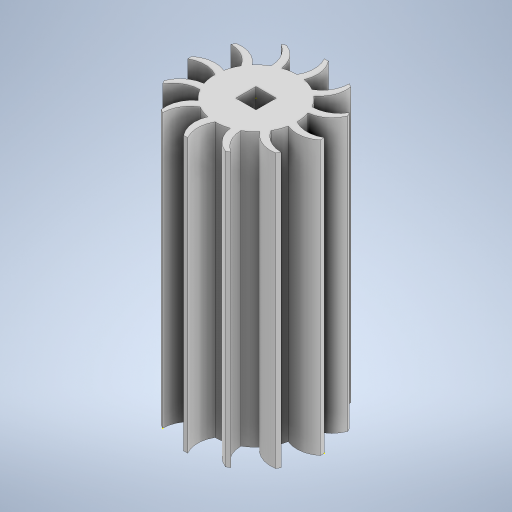
# Autodesk Inventor part: Part4
Saved by Autodesk Inventor 2023 (Build 270158000, 158)
## iProperties
Created: 2024-11-19
Part Number: Part4
Material: Generic
Document SubType Name: Sheet Metal
Designer: 1ZHUSAM
Density: 1 g/cm^3
Sheet Metal Rule: Default_mm
Appearance: Default
Author: 1ZHUSAM
Autodesk Inventor part; units mm, degrees
ref_plane "YZ Plane" through (0, 0, 0) normal (1, 0, 0) x (0, 1, 0)
ref_plane "XZ Plane" through (0, 0, 0) normal (0, 1, 0) x (-1, 0, 0)
ref_plane "XY Plane" through (0, 0, 0) normal (0, 0, 1) x (1, 0, 0)
sketch "Sketch1" plane through (0, 0, 0) normal (0, 1, 0) x (-1, 0, 0)
  circle A0 centre (0, 0) radius 7.5
  line L0 (1.5, 1.5) -> (-1.5, -1.5) construction
  line L1 (-1.5, 1.5) -> (1.5, -1.5) construction
  arc A1 (7.5, 0) -> (12.5, 0) centre (10, 4.3301) ccw
  line L2 (0, 0) -> (5.3033, -5.3033)
  line L3 (0, 0) -> (6.9291, -2.8701)
  line L4 (0, 0) -> (7.5, 0) construction
  line L5 (0, 0) -> (7.3559, -1.4632)
  line L6 (0, 0) -> (7.5, 0) construction
  line L7 (0, 0) -> (7.4639, -0.7351)
  line L8 (0, 0) -> (7.5, 0) construction
  line L9 (12.5, 0) -> (12.5, -0.7351)
  arc A2 (7.4639, -0.7351) -> (7.5, 0) centre (0, 0) ccw
  arc A3 (7.3559, -1.4632) -> (12.5, -0.7351) centre (9.3293, 3.1309) ccw
  arc A4 (6.4952, 3.75) -> (10.8253, 6.25) centre (6.4952, 8.75) ccw
  line L10 (10.8253, 6.25) -> (11.1929, 5.6134)
  arc A5 (7.102, 2.4108) -> (11.1929, 5.6134) centre (6.5139, 7.3761) ccw
  arc A6 (3.75, 6.4952) -> (6.25, 10.8253) centre (1.25, 10.8253) ccw
  line L11 (6.25, 10.8253) -> (6.8866, 10.4578)
  arc A7 (4.9451, 5.6388) -> (6.8866, 10.4578) centre (1.9532, 9.6448) ccw
  arc A8 (0, 7.5) -> (0, 12.5) centre (-4.3301, 10) ccw
  line L12 (0, 12.5) -> (0.7351, 12.5)
  arc A9 (1.4632, 7.3559) -> (0.7351, 12.5) centre (-3.1309, 9.3293) ccw
  arc A10 (-3.75, 6.4952) -> (-6.25, 10.8253) centre (-8.75, 6.4952) ccw
  line L13 (-6.25, 10.8253) -> (-5.6134, 11.1929)
  arc A11 (-2.4108, 7.102) -> (-5.6134, 11.1929) centre (-7.3761, 6.5139) ccw
  arc A12 (-6.4952, 3.75) -> (-10.8253, 6.25) centre (-10.8253, 1.25) ccw
  line L14 (-10.8253, 6.25) -> (-10.4578, 6.8866)
  arc A13 (-5.6388, 4.9451) -> (-10.4578, 6.8866) centre (-9.6448, 1.9532) ccw
  arc A14 (-7.5, 0) -> (-12.5, 0) centre (-10, -4.3301) ccw
  line L15 (-12.5, 0) -> (-12.5, 0.7351)
  arc A15 (-7.3559, 1.4632) -> (-12.5, 0.7351) centre (-9.3293, -3.1309) ccw
  arc A16 (-6.4952, -3.75) -> (-10.8253, -6.25) centre (-6.4952, -8.75) ccw
  line L16 (-10.8253, -6.25) -> (-11.1929, -5.6134)
  arc A17 (-7.102, -2.4108) -> (-11.1929, -5.6134) centre (-6.5139, -7.3761) ccw
  arc A18 (-3.75, -6.4952) -> (-6.25, -10.8253) centre (-1.25, -10.8253) ccw
  line L17 (-6.25, -10.8253) -> (-6.8866, -10.4578)
  arc A19 (-4.9451, -5.6388) -> (-6.8866, -10.4578) centre (-1.9532, -9.6448) ccw
  arc A20 (0, -7.5) -> (0, -12.5) centre (4.3301, -10) ccw
  line L18 (0, -12.5) -> (-0.7351, -12.5)
  arc A21 (-1.4632, -7.3559) -> (-0.7351, -12.5) centre (3.1309, -9.3293) ccw
  arc A22 (3.75, -6.4952) -> (6.25, -10.8253) centre (8.75, -6.4952) ccw
  line L19 (6.25, -10.8253) -> (5.6134, -11.1929)
  arc A23 (2.4108, -7.102) -> (5.6134, -11.1929) centre (7.3761, -6.5139) ccw
  arc A24 (6.4952, -3.75) -> (10.8253, -6.25) centre (10.8253, -1.25) ccw
  line L20 (10.8253, -6.25) -> (10.4578, -6.8866)
  arc A25 (5.6388, -4.9451) -> (10.4578, -6.8866) centre (9.6448, -1.9532) ccw
  line L21 (1.85, -1.85) -> (-1.85, -1.85)
  line L22 (-1.85, -1.85) -> (-1.85, 1.85)
  line L23 (-1.85, 1.85) -> (1.85, 1.85)
  line L24 (1.85, 1.85) -> (1.85, -1.85)
  line L25 (1.85, -1.85) -> (-1.85, 1.85) construction
  line L26 (-1.85, -1.85) -> (1.85, 1.85) construction
  point P0 (7.102, 2.4108)
  point P1 (6.4952, 3.75)
  point P2 (4.9451, 5.6388)
  point P3 (3.75, 6.4952)
  point P4 (1.4632, 7.3559)
  point P5 (0, 7.5)
  point P6 (-2.4108, 7.102)
  point P7 (-3.75, 6.4952)
  point P8 (-5.6388, 4.9451)
  point P9 (-6.4952, 3.75)
  point P10 (-7.3559, 1.4632)
  point P11 (-7.5, 0)
  point P12 (-1.4632, -7.3559)
  point P13 (0, -7.5)
  point P14 (2.4108, -7.102)
  point P15 (3.75, -6.4952)
  dimension "d0" = 15
  dimension "d1" = 3
  dimension "d2" = 3
  dimension "d3" = 5
  dimension "d4" = 5
  dimension "d5" = 22.5
  dimension "d6" = 11.25
  dimension "d7" = 5.625
  dimension "d13" = 5
  dimension "d16" = 360
  dimension "d20" = 3.7
  dimension "d21" = 3.7
  constraints: 54 end point, 50 point on circle, 25 centre point, 4 horizontal, 4 midpoint, 3 equal length, 2 parallel, 1 coincident, 1 perpendicular, 1 vertical, 117 other
  measures "d1" distance of L1.end L0.end
  measures "d2" distance of L0.end L1.start
  measures "d3" distance of A1.start L9.start
  measures "d4" radius of A1
  measures "d5" angle of L3 L4
  measures "d6" angle of L5 L6
  measures "d7" angle of L7 L8
  measures "d13" radius of A3
  measures "d20" distance of L22.end L23.end
  measures "d21" distance of L21.end L22.end
extrude "Extrusion1" add sketch "Sketch1" along normal blind 50 contours A0 L7 L24 L23 L22 L21 L2 | A1 L9 A3 A0 | A0 A4 L10 A5 | A0 L5 L24 L7 | A0 L3 L24 L5 | A0 A6 L11 A7 | A0 L2 L24 L3 | A24 L20 A25 A0 | A0 A8 L12 A9 | A22 L19 A23 A0 | A0 A10 L13 A11 | A20 L18 A21 A0 | A0 A12 L14 A13 | A18 L17 A19 A0 | A0 A14 L15 A15 | A16 L16 A17 A0
sketch "Sketch2" plane through (12.5, 0, 0) normal (1, 0, 0) x (0, 0, -1)
  point P0 (0, 0)
sketch "Sketch3" plane through (0, 50, 0) normal (0, 1, 0) x (1, 0, 0)
  point P0 (0, 0)
sketch "Sketch4" plane through (-6.25, 0, 10.8253) normal (-0.5, 0, 0.866) x (0.866, 0, 0.5)
  point P0 (0, 0)
sketch "Sketch5" plane through (0, 50, 0) normal (0, 1, 0) x (1, 0, 0)
  point P0 (0, 0)
equation "\"BendRadius\" = Thickness"
equation "\"BendReliefWidth\" = Thickness"
equation "\"BendReliefDepth\" = 0.5 * Thickness"
equation "\"CornerReliefSize\" = 4 * Thickness"
equation "\"MinimumRemnant\" = 2 * Thickness"
equation "\"TransitionRadius\" = BendRadius"
equation "\"JacobiRadiusSize\" = BendRadius"
equation "\"GapSize\" = Thickness"
equation "\"Thickness\" = 0.5"
body "Solid1"
